Autodesk Fusion 360 part; units mm, degrees
(part 5 of 6)
  arc A231 (-66.3069, 126.4592) -> (-66.9633, 126.6319) centre (-66.7286, 126.1905) ccw
  line L58 (-66.9633, 126.6319) -> (-67.5372, 126.3268)
  arc A232 (-67.5372, 126.3268) -> (-67.761, 125.686) centre (-67.3025, 125.8853) ccw
  arc A233 (-68.3566, 123.3185) -> (-67.761, 125.686) centre (-69.5953, 124.8887) ccw
  arc A234 (-70.6799, 124.068) -> (-68.3566, 123.3185) centre (-69.0318, 125.2011) ccw
  arc A235 (-70.6799, 124.068) -> (-71.3419, 124.2178) centre (-71.0919, 123.7848) ccw
  line L59 (-71.3419, 124.2178) -> (-71.9048, 123.8928)
  arc A236 (-71.9048, 123.8928) -> (-72.1061, 123.2446) centre (-71.6548, 123.4598) ccw
  arc A237 (-72.6187, 120.8578) -> (-72.1061, 123.2446) centre (-73.9114, 122.3838) ccw
  arc A238 (-74.9667, 121.5258) -> (-72.6187, 120.8578) centre (-73.3592, 122.7156) ccw
  arc A239 (-74.9667, 121.5258) -> (-75.6336, 121.6523) centre (-75.3686, 121.2283) ccw
  line L60 (-75.6336, 121.6523) -> (-76.1848, 121.3079)
  arc A240 (-76.1848, 121.3079) -> (-76.3634, 120.653) centre (-75.9199, 120.8839) ccw
  arc A241 (-76.7923, 118.2498) -> (-76.3634, 120.653) centre (-78.1375, 119.7298) ccw
  arc A242 (-79.1623, 118.8354) -> (-76.7923, 118.2498) centre (-77.5972, 120.0807) ccw
  arc A243 (-79.1623, 118.8354) -> (-79.8331, 118.9387) centre (-79.5535, 118.5241) ccw
  line L61 (-79.8331, 118.9387) -> (-80.372, 118.5752)
  arc A244 (-80.372, 118.5752) -> (-80.5276, 117.9145) centre (-80.0924, 118.1607) ccw
  arc A245 (-80.8724, 115.4978) -> (-80.5276, 117.9145) centre (-82.2684, 116.9299) ccw
  arc A246 (-83.2613, 116.0003) -> (-80.8724, 115.4978) centre (-81.7407, 117.2994) ccw
  arc A247 (-83.2613, 116.0003) -> (-83.9354, 116.0801) centre (-83.6415, 115.6756) ccw
  line L62 (-83.9354, 116.0801) -> (-84.4612, 115.698)
  arc A248 (-84.4612, 115.698) -> (-84.5937, 115.0323) centre (-84.1673, 115.2935) ccw
  arc A249 (-84.8539, 112.605) -> (-84.5937, 115.0323) centre (-86.2991, 113.9875) ccw
  arc A250 (-87.259, 113.0239) -> (-84.8539, 112.605) centre (-85.7846, 114.3753) ccw
  arc A251 (-87.259, 113.0239) -> (-87.9354, 113.08) centre (-87.6276, 112.686) ccw
  line L63 (-87.9354, 113.08) -> (-88.4476, 112.6799)
  arc A252 (-88.4476, 112.6799) -> (-88.5567, 112.01) centre (-88.1398, 112.2859) ccw
  arc A253 (-88.7321, 109.575) -> (-88.5567, 112.01) centre (-90.2247, 110.9063) ccw
  arc A254 (-91.1503, 109.9097) -> (-88.7321, 109.575) centre (-89.724, 111.3118) ccw
  arc A255 (-91.1503, 109.9097) -> (-91.8283, 109.9423) centre (-91.5069, 109.5592) ccw
  line L64 (-91.8283, 109.9423) -> (-92.3262, 109.5244)
  arc A256 (-92.3262, 109.5244) -> (-92.4119, 108.8511) centre (-92.0048, 109.1414) ccw
  arc A257 (-92.5022, 106.4116) -> (-92.4119, 108.8511) centre (-94.0403, 107.6899) ccw
  arc A258 (-94.9306, 106.6617) -> (-92.5022, 106.4116) centre (-93.554, 108.1126) ccw
  arc A259 (-94.9306, 106.6617) -> (-95.6092, 106.6705) centre (-95.2747, 106.299) ccw
  line L65 (-95.6092, 106.6705) -> (-96.0923, 106.2356)
  arc A260 (-96.0923, 106.2356) -> (-96.1544, 105.5597) centre (-95.7577, 105.864) ccw
  arc A261 (-96.1595, 103.1185) -> (-96.1544, 105.5597) centre (-97.7413, 104.3424) ccw
  arc A262 (-98.5952, 103.2837) -> (-96.1595, 103.1185) centre (-97.2701, 104.7818) ccw
  arc A263 (-98.5952, 103.2837) -> (-99.2737, 103.2688) centre (-98.9264, 102.9092) ccw
  line L66 (-99.2737, 103.2688) -> (-99.7413, 102.8173)
  arc A264 (-99.7413, 102.8173) -> (-99.7798, 102.1396) centre (-99.394, 102.4576) ccw
  arc A265 (-99.6997, 99.6997) -> (-99.7798, 102.1396) centre (-101.3233, 100.8677) ccw
  arc A266 (-102.1396, 99.7798) -> (-99.6997, 99.6997) centre (-100.8677, 101.3233) ccw
  arc A267 (-102.1396, 99.7798) -> (-102.8173, 99.7413) centre (-102.4576, 99.394) ccw
  line L67 (-102.8173, 99.7413) -> (-103.2688, 99.2737)
  arc A268 (-103.2688, 99.2737) -> (-103.2837, 98.5952) centre (-102.9092, 98.9264) ccw
  arc A269 (-103.1185, 96.1595) -> (-103.2837, 98.5952) centre (-104.7818, 97.2701) ccw
  arc A270 (-105.5597, 96.1544) -> (-103.1185, 96.1595) centre (-104.3424, 97.7413) ccw
  arc A271 (-105.5597, 96.1544) -> (-106.2356, 96.0923) centre (-105.864, 95.7577) ccw
  line L68 (-106.2356, 96.0923) -> (-106.6705, 95.6092)
  arc A272 (-106.6705, 95.6092) -> (-106.6617, 94.9306) centre (-106.299, 95.2747) ccw
  arc A273 (-106.4116, 92.5022) -> (-106.6617, 94.9306) centre (-108.1126, 93.554) ccw
  arc A274 (-108.8511, 92.4119) -> (-106.4116, 92.5022) centre (-107.6899, 94.0403) ccw
  arc A275 (-108.8511, 92.4119) -> (-109.5244, 92.3262) centre (-109.1414, 92.0048) ccw
  line L69 (-109.5244, 92.3262) -> (-109.9423, 91.8283)
  arc A276 (-109.9423, 91.8283) -> (-109.9097, 91.1503) centre (-109.5592, 91.5069) ccw
  arc A277 (-109.575, 88.7321) -> (-109.9097, 91.1503) centre (-111.3118, 89.724) ccw
  arc A278 (-112.01, 88.5567) -> (-109.575, 88.7321) centre (-110.9063, 90.2247) ccw
  arc A279 (-112.01, 88.5567) -> (-112.6799, 88.4476) centre (-112.2859, 88.1398) ccw
  line L70 (-112.6799, 88.4476) -> (-113.08, 87.9354)
  arc A280 (-113.08, 87.9354) -> (-113.0239, 87.259) centre (-112.686, 87.6276) ccw
  arc A281 (-112.605, 84.8539) -> (-113.0239, 87.259) centre (-114.3753, 85.7846) ccw
  arc A282 (-115.0323, 84.5937) -> (-112.605, 84.8539) centre (-113.9875, 86.2991) ccw
  arc A283 (-115.0323, 84.5937) -> (-115.698, 84.4612) centre (-115.2935, 84.1673) ccw
  line L71 (-115.698, 84.4612) -> (-116.0801, 83.9354)
  arc A284 (-116.0801, 83.9354) -> (-116.0003, 83.2613) centre (-115.6756, 83.6415) ccw
  arc A285 (-115.4978, 80.8724) -> (-116.0003, 83.2613) centre (-117.2994, 81.7407) ccw
  arc A286 (-117.9145, 80.5276) -> (-115.4978, 80.8724) centre (-116.9299, 82.2684) ccw
  arc A287 (-117.9145, 80.5276) -> (-118.5752, 80.372) centre (-118.1607, 80.0924) ccw
  line L72 (-118.5752, 80.372) -> (-118.9387, 79.8331)
  arc A288 (-118.9387, 79.8331) -> (-118.8354, 79.1623) centre (-118.5241, 79.5535) ccw
  arc A289 (-118.2498, 76.7923) -> (-118.8354, 79.1623) centre (-120.0807, 77.5972) ccw
  arc A290 (-120.653, 76.3634) -> (-118.2498, 76.7923) centre (-119.7298, 78.1375) ccw
  arc A291 (-120.653, 76.3634) -> (-121.3079, 76.1848) centre (-120.8839, 75.9199) ccw
  line L73 (-121.3079, 76.1848) -> (-121.6523, 75.6336)
  arc A292 (-121.6523, 75.6336) -> (-121.5258, 74.9667) centre (-121.2283, 75.3686) ccw
  arc A293 (-120.8578, 72.6187) -> (-121.5258, 74.9667) centre (-122.7156, 73.3592) ccw
  arc A294 (-123.2446, 72.1061) -> (-120.8578, 72.6187) centre (-122.3838, 73.9114) ccw
  arc A295 (-123.2446, 72.1061) -> (-123.8928, 71.9048) centre (-123.4598, 71.6548) ccw
  line L74 (-123.8928, 71.9048) -> (-124.2178, 71.3419)
  arc A296 (-124.2178, 71.3419) -> (-124.068, 70.6799) centre (-123.7848, 71.0919) ccw
  arc A297 (-123.3185, 68.3566) -> (-124.068, 70.6799) centre (-125.2011, 69.0318) ccw
  arc A298 (-125.686, 67.761) -> (-123.3185, 68.3566) centre (-124.8887, 69.5953) ccw
  arc A299 (-125.686, 67.761) -> (-126.3268, 67.5372) centre (-125.8853, 67.3025) ccw
  line L75 (-126.3268, 67.5372) -> (-126.6319, 66.9633)
  arc A300 (-126.6319, 66.9633) -> (-126.4592, 66.3069) centre (-126.1905, 66.7286) ccw
  arc A301 (-125.629, 64.0112) -> (-126.4592, 66.3069) centre (-127.534, 64.6203) ccw
  arc A302 (-127.9742, 63.3334) -> (-125.629, 64.0112) centre (-127.2415, 65.1943) ccw
  arc A303 (-127.9742, 63.3334) -> (-128.6068, 63.0873) centre (-128.1574, 62.8682) ccw
  line L76 (-128.6068, 63.0873) -> (-128.8918, 62.5031)
  arc A304 (-128.8918, 62.5031) -> (-128.6962, 61.8532) centre (-128.4424, 62.2839) ccw
  arc A305 (-127.7864, 59.5878) -> (-128.6962, 61.8532) centre (-129.7115, 60.13) ccw
  arc A306 (-130.1066, 58.8286) -> (-127.7864, 59.5878) centre (-129.4392, 60.7139) ccw
  arc A307 (-130.1066, 58.8286) -> (-130.7302, 58.5606) centre (-130.2734, 58.3572) ccw
  line L77 (-130.7302, 58.5606) -> (-130.9946, 57.9668)
  arc A308 (-130.9946, 57.9668) -> (-130.7764, 57.324) centre (-130.5378, 57.7634) ccw
  arc A309 (-129.7882, 55.0918) -> (-130.7764, 57.324) centre (-131.731, 55.5665) ccw
  arc A310 (-132.0804, 54.2521) -> (-129.7882, 55.0918) centre (-131.4793, 56.1596) ccw
  arc A311 (-132.0804, 54.2521) -> (-132.6943, 53.9625) centre (-132.2307, 53.7752) ccw
  line L78 (-132.6943, 53.9625) -> (-132.9378, 53.3598)
  arc A312 (-132.9378, 53.3598) -> (-132.6974, 52.7251) centre (-132.4742, 53.1725) ccw
  arc A313 (-131.6318, 50.5287) -> (-132.6974, 52.7251) centre (-133.59, 50.9353) ccw
  arc A314 (-133.8933, 49.6095) -> (-131.6318, 50.5287) centre (-133.3591, 51.5368) ccw
  arc A315 (-133.8933, 49.6095) -> (-134.4967, 49.2987) centre (-134.0269, 49.1277) ccw
  line L79 (-134.4967, 49.2987) -> (-134.719, 48.6879)
  arc A316 (-134.719, 48.6879) -> (-134.4566, 48.0619) centre (-134.2492, 48.5169) ccw
  arc A317 (-133.315, 45.904) -> (-134.4566, 48.0619) centre (-135.2862, 46.2421) ccw
  arc A318 (-135.5431, 44.9065) -> (-133.315, 45.904) centre (-135.0765, 46.8513) ccw
  arc A319 (-135.5431, 44.9065) -> (-136.1353, 44.5748) centre (-135.6598, 44.4203) ccw
  line L80 (-136.1353, 44.5748) -> (-136.3362, 43.9566)
  arc A320 (-136.3362, 43.9566) -> (-136.052, 43.3402) centre (-135.8606, 43.8021) ccw
  arc A321 (-134.8358, 41.2235) -> (-136.052, 43.3402) centre (-136.8177, 41.4925) ccw
  arc A322 (-137.0278, 40.1487) -> (-134.8358, 41.2235) centre (-136.6293, 42.1086) ccw
  arc A323 (-137.0278, 40.1487) -> (-137.608, 39.7966) centre (-137.1274, 39.6587) ccw
  line L81 (-137.608, 39.7966) -> (-137.7872, 39.1717)
  arc A324 (-137.7872, 39.1717) -> (-137.4817, 38.5656) centre (-137.3065, 39.0339) ccw
  arc A325 (-136.1924, 36.4926) -> (-137.4817, 38.5656) centre (-138.1824, 36.6924) ccw
  arc A326 (-138.3455, 35.3421) -> (-136.1924, 36.4926) centre (-138.0156, 37.3147) ccw
  arc A327 (-138.3455, 35.3421) -> (-138.9131, 34.9699) centre (-138.4279, 34.8489) ccw
  line L82 (-138.9131, 34.9699) -> (-139.0703, 34.3392)
  arc A328 (-139.0703, 34.3392) -> (-138.7439, 33.7441) centre (-138.5852, 34.2182) ccw
  arc A329 (-137.383, 31.7174) -> (-138.7439, 33.7441) centre (-139.3787, 31.8475) ccw
  arc A330 (-139.4946, 30.4923) -> (-137.383, 31.7174) centre (-139.2338, 32.4753) ccw
  arc A331 (-139.4946, 30.4923) -> (-140.0489, 30.1006) centre (-139.5598, 29.9966) ccw
  line L83 (-140.0489, 30.1006) -> (-140.184, 29.4648)
  arc A332 (-140.184, 29.4648) -> (-139.837, 28.8814) centre (-139.6949, 29.3608) ccw
  arc A333 (-138.4062, 26.9034) -> (-139.837, 28.8814) centre (-140.4053, 26.9639) ccw
  arc A334 (-140.4738, 25.6055) -> (-138.4062, 26.9034) centre (-140.2824, 27.5963) ccw
  arc A335 (-140.4738, 25.6055) -> (-141.014, 25.1946) centre (-140.5216, 25.1078) ccw
  line L84 (-141.014, 25.1946) -> (-141.1269, 24.5545)
  arc A336 (-141.1269, 24.5545) -> (-140.7598, 23.9836) centre (-140.6345, 24.4676) ccw
  arc A337 (-139.2608, 22.0567) -> (-140.7598, 23.9836) centre (-141.2608, 22.0474) ccw
  arc A338 (-141.2818, 20.6874) -> (-139.2608, 22.0567) centre (-141.16, 22.6837) ccw
  arc A339 (-141.2818, 20.6874) -> (-141.8074, 20.2579) centre (-141.3123, 20.1883) ccw
  line L85 (-141.8074, 20.2579) -> (-141.8979, 19.6143)
  arc A340 (-141.8979, 19.6143) -> (-141.511, 19.0565) centre (-141.4028, 19.5447) ccw
  arc A341 (-139.9458, 17.1832) -> (-141.511, 19.0565) centre (-141.9442, 17.104) ccw
  arc A342 (-141.9177, 15.7441) -> (-139.9458, 17.1832) centre (-141.8657, 17.7435) ccw
  arc A343 (-141.9177, 15.7441) -> (-142.428, 15.2966) centre (-141.9308, 15.2443) ccw
  line L86 (-142.428, 15.2966) -> (-142.496, 14.6501)
  arc A344 (-142.496, 14.6501) -> (-142.0899, 14.1063) centre (-141.9987, 14.5979) ccw
  arc A345 (-140.4602, 12.2887) -> (-142.0899, 14.1063) centre (-142.4546, 12.1398) ccw
  arc A346 (-142.3808, 10.7817) -> (-140.4602, 12.2887) centre (-142.3985, 12.7816) ccw
  arc A347 (-142.3808, 10.7817) -> (-142.8751, 10.3166) centre (-142.3763, 10.2817) ccw
  line L87 (-142.8751, 10.3166) -> (-142.9205, 9.6682)
  arc A348 (-142.9205, 9.6682) -> (-142.4956, 9.1388) centre (-142.4217, 9.6333) ccw
  arc A349 (-140.8035, 7.3792) -> (-142.4956, 9.1388) centre (-142.7915, 7.1608) ccw
  arc A350 (-142.6703, 5.8061) -> (-140.8035, 7.3792) centre (-142.7578, 7.8042) ccw
  arc A351 (-142.6703, 5.8061) -> (-143.1481, 5.324) centre (-142.6484, 5.3066) ccw
  line L88 (-143.1481, 5.324) -> (-143.1708, 4.6744)
  arc A352 (-143.1708, 4.6744) -> (-142.7278, 4.1602) centre (-142.6711, 4.657) ccw
  arc A353 (-140.9752, 2.4607) -> (-142.7278, 4.1602) centre (-142.9545, 2.1731) ccw
  arc A354 (-142.786, 0.8235) -> (-140.9752, 2.4607) centre (-142.9432, 2.8173) ccw
  arc A355 (-142.786, 0.8235) -> (-143.2467, 0.325) centre (-142.7467, 0.325) ccw
  line L89 (-143.2467, 0.325) -> (-143.2467, -0.325)
  arc A356 (-143.2467, -0.325) -> (-142.786, -0.8235) centre (-142.7467, -0.325) ccw
  arc A357 (-140.9752, -2.4607) -> (-142.786, -0.8235) centre (-142.9432, -2.8173) ccw
  arc A358 (-142.7278, -4.1602) -> (-140.9752, -2.4607) centre (-142.9545, -2.1731) ccw
  arc A359 (-142.7278, -4.1602) -> (-143.1708, -4.6744) centre (-142.6711, -4.657) ccw
  line L90 (-143.1708, -4.6744) -> (-143.1481, -5.324)
  arc A360 (-143.1481, -5.324) -> (-142.6703, -5.8061) centre (-142.6484, -5.3066) ccw
  arc A361 (-140.8035, -7.3792) -> (-142.6703, -5.8061) centre (-142.7578, -7.8042) ccw
  arc A362 (-142.4956, -9.1388) -> (-140.8035, -7.3792) centre (-142.7915, -7.1608) ccw
  arc A363 (-142.4956, -9.1388) -> (-142.9205, -9.6682) centre (-142.4217, -9.6333) ccw
  line L91 (-142.9205, -9.6682) -> (-142.8751, -10.3166)
  arc A364 (-142.8751, -10.3166) -> (-142.3808, -10.7817) centre (-142.3763, -10.2817) ccw
  arc A365 (-140.4602, -12.2887) -> (-142.3808, -10.7817) centre (-142.3985, -12.7816) ccw
  arc A366 (-142.0899, -14.1063) -> (-140.4602, -12.2887) centre (-142.4546, -12.1398) ccw
  arc A367 (-142.0899, -14.1063) -> (-142.496, -14.6501) centre (-141.9987, -14.5979) ccw
  line L92 (-142.496, -14.6501) -> (-142.428, -15.2966)
  arc A368 (-142.428, -15.2966) -> (-141.9177, -15.7441) centre (-141.9308, -15.2443) ccw
  arc A369 (-139.9458, -17.1832) -> (-141.9177, -15.7441) centre (-141.8657, -17.7435) ccw
  arc A370 (-141.511, -19.0565) -> (-139.9458, -17.1832) centre (-141.9442, -17.104) ccw
  arc A371 (-141.511, -19.0565) -> (-141.8979, -19.6143) centre (-141.4028, -19.5447) ccw
  line L93 (-141.8979, -19.6143) -> (-141.8074, -20.2579)
  arc A372 (-141.8074, -20.2579) -> (-141.2818, -20.6874) centre (-141.3123, -20.1883) ccw
  arc A373 (-139.2608, -22.0567) -> (-141.2818, -20.6874) centre (-141.16, -22.6837) ccw
  arc A374 (-140.7598, -23.9836) -> (-139.2608, -22.0567) centre (-141.2608, -22.0474) ccw
  arc A375 (-140.7598, -23.9836) -> (-141.1269, -24.5545) centre (-140.6345, -24.4676) ccw
  line L94 (-141.1269, -24.5545) -> (-141.014, -25.1946)
  arc A376 (-141.014, -25.1946) -> (-140.4738, -25.6055) centre (-140.5216, -25.1078) ccw
  arc A377 (-138.4062, -26.9034) -> (-140.4738, -25.6055) centre (-140.2824, -27.5963) ccw
  arc A378 (-139.837, -28.8814) -> (-138.4062, -26.9034) centre (-140.4053, -26.9639) ccw
  arc A379 (-139.837, -28.8814) -> (-140.184, -29.4648) centre (-139.6949, -29.3608) ccw
  line L95 (-140.184, -29.4648) -> (-140.0489, -30.1006)
  arc A380 (-140.0489, -30.1006) -> (-139.4946, -30.4923) centre (-139.5598, -29.9966) ccw
  arc A381 (-137.383, -31.7174) -> (-139.4946, -30.4923) centre (-139.2338, -32.4753) ccw
  arc A382 (-138.7439, -33.7441) -> (-137.383, -31.7174) centre (-139.3787, -31.8475) ccw
  arc A383 (-138.7439, -33.7441) -> (-139.0703, -34.3392) centre (-138.5852, -34.2182) ccw
  line L96 (-139.0703, -34.3392) -> (-138.9131, -34.9699)
  arc A384 (-138.9131, -34.9699) -> (-138.3455, -35.3421) centre (-138.4279, -34.8489) ccw
  arc A385 (-136.1924, -36.4926) -> (-138.3455, -35.3421) centre (-138.0156, -37.3147) ccw
  arc A386 (-137.4817, -38.5656) -> (-136.1924, -36.4926) centre (-138.1824, -36.6924) ccw
  arc A387 (-137.4817, -38.5656) -> (-137.7872, -39.1717) centre (-137.3065, -39.0339) ccw
  line L97 (-137.7872, -39.1717) -> (-137.608, -39.7966)
  arc A388 (-137.608, -39.7966) -> (-137.0278, -40.1487) centre (-137.1274, -39.6587) ccw
  arc A389 (-134.8358, -41.2235) -> (-137.0278, -40.1487) centre (-136.6293, -42.1086) ccw
  arc A390 (-136.052, -43.3402) -> (-134.8358, -41.2235) centre (-136.8177, -41.4925) ccw
  arc A391 (-136.052, -43.3402) -> (-136.3362, -43.9566) centre (-135.8606, -43.8021) ccw
  line L98 (-136.3362, -43.9566) -> (-136.1353, -44.5748)
  arc A392 (-136.1353, -44.5748) -> (-135.5431, -44.9065) centre (-135.6598, -44.4203) ccw
  arc A393 (-133.315, -45.904) -> (-135.5431, -44.9065) centre (-135.0765, -46.8513) ccw
  arc A394 (-134.4566, -48.0619) -> (-133.315, -45.904) centre (-135.2862, -46.2421) ccw
  arc A395 (-134.4566, -48.0619) -> (-134.719, -48.6879) centre (-134.2492, -48.5169) ccw
  line L99 (-134.719, -48.6879) -> (-134.4967, -49.2987)
  arc A396 (-134.4967, -49.2987) -> (-133.8933, -49.6095) centre (-134.0269, -49.1277) ccw
  arc A397 (-131.6318, -50.5287) -> (-133.8933, -49.6095) centre (-133.3591, -51.5368) ccw
  arc A398 (-132.6974, -52.7251) -> (-131.6318, -50.5287) centre (-133.59, -50.9353) ccw
  arc A399 (-132.6974, -52.7251) -> (-132.9378, -53.3598) centre (-132.4742, -53.1725) ccw
  line L100 (-132.9378, -53.3598) -> (-132.6943, -53.9625)
  arc A400 (-132.6943, -53.9625) -> (-132.0804, -54.2521) centre (-132.2307, -53.7752) ccw
  arc A401 (-129.7882, -55.0918) -> (-132.0804, -54.2521) centre (-131.4793, -56.1596) ccw
  arc A402 (-130.7764, -57.324) -> (-129.7882, -55.0918) centre (-131.731, -55.5665) ccw
  arc A403 (-130.7764, -57.324) -> (-130.9946, -57.9668) centre (-130.5378, -57.7634) ccw
  line L101 (-130.9946, -57.9668) -> (-130.7302, -58.5606)
  arc A404 (-130.7302, -58.5606) -> (-130.1066, -58.8286) centre (-130.2734, -58.3572) ccw
  arc A405 (-127.7864, -59.5878) -> (-130.1066, -58.8286) centre (-129.4392, -60.7139) ccw
  arc A406 (-128.6962, -61.8532) -> (-127.7864, -59.5878) centre (-129.7115, -60.13) ccw
  arc A407 (-128.6962, -61.8532) -> (-128.8918, -62.5031) centre (-128.4424, -62.2839) ccw
  line L102 (-128.8918, -62.5031) -> (-128.6068, -63.0873)
  arc A408 (-128.6068, -63.0873) -> (-127.9742, -63.3334) centre (-128.1574, -62.8682) ccw
  arc A409 (-125.629, -64.0112) -> (-127.9742, -63.3334) centre (-127.2415, -65.1943) ccw
  arc A410 (-126.4592, -66.3069) -> (-125.629, -64.0112) centre (-127.534, -64.6203) ccw
  arc A411 (-126.4592, -66.3069) -> (-126.6319, -66.9633) centre (-126.1905, -66.7286) ccw
  line L103 (-126.6319, -66.9633) -> (-126.3268, -67.5372)
  arc A412 (-126.3268, -67.5372) -> (-125.686, -67.761) centre (-125.8853, -67.3025) ccw
  arc A413 (-123.3185, -68.3566) -> (-125.686, -67.761) centre (-124.8887, -69.5953) ccw
  arc A414 (-124.068, -70.6799) -> (-123.3185, -68.3566) centre (-125.2011, -69.0318) ccw
  arc A415 (-124.068, -70.6799) -> (-124.2178, -71.3419) centre (-123.7848, -71.0919) ccw
  line L104 (-124.2178, -71.3419) -> (-123.8928, -71.9048)
  arc A416 (-123.8928, -71.9048) -> (-123.2446, -72.1061) centre (-123.4598, -71.6548) ccw
  arc A417 (-120.8578, -72.6187) -> (-123.2446, -72.1061) centre (-122.3838, -73.9114) ccw
  arc A418 (-121.5258, -74.9667) -> (-120.8578, -72.6187) centre (-122.7156, -73.3592) ccw
  arc A419 (-121.5258, -74.9667) -> (-121.6523, -75.6336) centre (-121.2283, -75.3686) ccw
  line L105 (-121.6523, -75.6336) -> (-121.3079, -76.1848)
  arc A420 (-121.3079, -76.1848) -> (-120.653, -76.3634) centre (-120.8839, -75.9199) ccw
  arc A421 (-118.2498, -76.7923) -> (-120.653, -76.3634) centre (-119.7298, -78.1375) ccw
  arc A422 (-118.8354, -79.1623) -> (-118.2498, -76.7923) centre (-120.0807, -77.5972) ccw
  arc A423 (-118.8354, -79.1623) -> (-118.9387, -79.8331) centre (-118.5241, -79.5535) ccw
  line L106 (-118.9387, -79.8331) -> (-118.5752, -80.372)
  arc A424 (-118.5752, -80.372) -> (-117.9145, -80.5276) centre (-118.1607, -80.0924) ccw
  arc A425 (-115.4978, -80.8724) -> (-117.9145, -80.5276) centre (-116.9299, -82.2684) ccw
  arc A426 (-116.0003, -83.2613) -> (-115.4978, -80.8724) centre (-117.2994, -81.7407) ccw
  arc A427 (-116.0003, -83.2613) -> (-116.0801, -83.9354) centre (-115.6756, -83.6415) ccw
  line L107 (-116.0801, -83.9354) -> (-115.698, -84.4612)
  arc A428 (-115.698, -84.4612) -> (-115.0323, -84.5937) centre (-115.2935, -84.1673) ccw
  arc A429 (-112.605, -84.8539) -> (-115.0323, -84.5937) centre (-113.9875, -86.2991) ccw
  arc A430 (-113.0239, -87.259) -> (-112.605, -84.8539) centre (-114.3753, -85.7846) ccw
  arc A431 (-113.0239, -87.259) -> (-113.08, -87.9354) centre (-112.686, -87.6276) ccw
  line L108 (-113.08, -87.9354) -> (-112.6799, -88.4476)
  arc A432 (-112.6799, -88.4476) -> (-112.01, -88.5567) centre (-112.2859, -88.1398) ccw
  arc A433 (-109.575, -88.7321) -> (-112.01, -88.5567) centre (-110.9063, -90.2247) ccw
  arc A434 (-109.9097, -91.1503) -> (-109.575, -88.7321) centre (-111.3118, -89.724) ccw
  arc A435 (-109.9097, -91.1503) -> (-109.9423, -91.8283) centre (-109.5592, -91.5069) ccw
  line L109 (-109.9423, -91.8283) -> (-109.5244, -92.3262)
  arc A436 (-109.5244, -92.3262) -> (-108.8511, -92.4119) centre (-109.1414, -92.0048) ccw
  arc A437 (-106.4116, -92.5022) -> (-108.8511, -92.4119) centre (-107.6899, -94.0403) ccw
  arc A438 (-106.6617, -94.9306) -> (-106.4116, -92.5022) centre (-108.1126, -93.554) ccw
  arc A439 (-106.6617, -94.9306) -> (-106.6705, -95.6092) centre (-106.299, -95.2747) ccw
  line L110 (-106.6705, -95.6092) -> (-106.2356, -96.0923)
  arc A440 (-106.2356, -96.0923) -> (-105.5597, -96.1544) centre (-105.864, -95.7577) ccw
  arc A441 (-103.1185, -96.1595) -> (-105.5597, -96.1544) centre (-104.3424, -97.7413) ccw
  arc A442 (-103.2837, -98.5952) -> (-103.1185, -96.1595) centre (-104.7818, -97.2701) ccw
  arc A443 (-103.2837, -98.5952) -> (-103.2688, -99.2737) centre (-102.9092, -98.9264) ccw
  line L111 (-103.2688, -99.2737) -> (-102.8173, -99.7413)
  arc A444 (-102.8173, -99.7413) -> (-102.1396, -99.7798) centre (-102.4576, -99.394) ccw
  arc A445 (-99.6997, -99.6997) -> (-102.1396, -99.7798) centre (-100.8677, -101.3233) ccw
  arc A446 (-99.7798, -102.1396) -> (-99.6997, -99.6997) centre (-101.3233, -100.8677) ccw
  arc A447 (-99.7798, -102.1396) -> (-99.7413, -102.8173) centre (-99.394, -102.4576) ccw
  line L112 (-99.7413, -102.8173) -> (-99.2737, -103.2688)
  arc A448 (-99.2737, -103.2688) -> (-98.5952, -103.2837) centre (-98.9264, -102.9092) ccw
  arc A449 (-96.1595, -103.1185) -> (-98.5952, -103.2837) centre (-97.2701, -104.7818) ccw
  arc A450 (-96.1544, -105.5597) -> (-96.1595, -103.1185) centre (-97.7413, -104.3424) ccw
  arc A451 (-96.1544, -105.5597) -> (-96.0923, -106.2356) centre (-95.7577, -105.864) ccw
  line L113 (-96.0923, -106.2356) -> (-95.6092, -106.6705)
  arc A452 (-95.6092, -106.6705) -> (-94.9306, -106.6617) centre (-95.2747, -106.299) ccw
  arc A453 (-92.5022, -106.4116) -> (-94.9306, -106.6617) centre (-93.554, -108.1126) ccw
  arc A454 (-92.4119, -108.8511) -> (-92.5022, -106.4116) centre (-94.0403, -107.6899) ccw
  arc A455 (-92.4119, -108.8511) -> (-92.3262, -109.5244) centre (-92.0048, -109.1414) ccw
  line L114 (-92.3262, -109.5244) -> (-91.8283, -109.9423)
  arc A456 (-91.8283, -109.9423) -> (-91.1503, -109.9097) centre (-91.5069, -109.5592) ccw
  arc A457 (-88.7321, -109.575) -> (-91.1503, -109.9097) centre (-89.724, -111.3118) ccw
  arc A458 (-88.5567, -112.01) -> (-88.7321, -109.575) centre (-90.2247, -110.9063) ccw
  arc A459 (-88.5567, -112.01) -> (-88.4476, -112.6799) centre (-88.1398, -112.2859) ccw
  line L115 (-88.4476, -112.6799) -> (-87.9354, -113.08)
  arc A460 (-87.9354, -113.08) -> (-87.259, -113.0239) centre (-87.6276, -112.686) ccw
  arc A461 (-84.8539, -112.605) -> (-87.259, -113.0239) centre (-85.7846, -114.3753) ccw
  arc A462 (-84.5937, -115.0323) -> (-84.8539, -112.605) centre (-86.2991, -113.9875) ccw
  arc A463 (-84.5937, -115.0323) -> (-84.4612, -115.698) centre (-84.1673, -115.2935) ccw
  line L116 (-84.4612, -115.698) -> (-83.9354, -116.0801)
  arc A464 (-83.9354, -116.0801) -> (-83.2613, -116.0003) centre (-83.6415, -115.6756) ccw
  arc A465 (-80.8724, -115.4978) -> (-83.2613, -116.0003) centre (-81.7407, -117.2994) ccw
  arc A466 (-80.5276, -117.9145) -> (-80.8724, -115.4978) centre (-82.2684, -116.9299) ccw
  arc A467 (-80.5276, -117.9145) -> (-80.372, -118.5752) centre (-80.0924, -118.1607) ccw
  line L117 (-80.372, -118.5752) -> (-79.8331, -118.9387)
  arc A468 (-79.8331, -118.9387) -> (-79.1623, -118.8354) centre (-79.5535, -118.5241) ccw
  arc A469 (-76.7923, -118.2498) -> (-79.1623, -118.8354) centre (-77.5972, -120.0807) ccw
  arc A470 (-76.3634, -120.653) -> (-76.7923, -118.2498) centre (-78.1375, -119.7298) ccw
  arc A471 (-76.3634, -120.653) -> (-76.1848, -121.3079) centre (-75.9199, -120.8839) ccw
  line L118 (-76.1848, -121.3079) -> (-75.6336, -121.6523)
  arc A472 (-75.6336, -121.6523) -> (-74.9667, -121.5258) centre (-75.3686, -121.2283) ccw
  arc A473 (-72.6187, -120.8578) -> (-74.9667, -121.5258) centre (-73.3592, -122.7156) ccw
  arc A474 (-72.1061, -123.2446) -> (-72.6187, -120.8578) centre (-73.9114, -122.3838) ccw
  arc A475 (-72.1061, -123.2446) -> (-71.9048, -123.8928) centre (-71.6548, -123.4598) ccw
  line L119 (-71.9048, -123.8928) -> (-71.3419, -124.2178)
  arc A476 (-71.3419, -124.2178) -> (-70.6799, -124.068) centre (-71.0919, -123.7848) ccw
  arc A477 (-68.3566, -123.3185) -> (-70.6799, -124.068) centre (-69.0318, -125.2011) ccw
  arc A478 (-67.761, -125.686) -> (-68.3566, -123.3185) centre (-69.5953, -124.8887) ccw
  arc A479 (-67.761, -125.686) -> (-67.5372, -126.3268) centre (-67.3025, -125.8853) ccw
  line L120 (-67.5372, -126.3268) -> (-66.9633, -126.6319)
  arc A480 (-66.9633, -126.6319) -> (-66.3069, -126.4592) centre (-66.7286, -126.1905) ccw
  arc A481 (-64.0112, -125.629) -> (-66.3069, -126.4592) centre (-64.6203, -127.534) ccw
  arc A482 (-63.3334, -127.9742) -> (-64.0112, -125.629) centre (-65.1943, -127.2415) ccw
  arc A483 (-63.3334, -127.9742) -> (-63.0873, -128.6068) centre (-62.8682, -128.1574) ccw
  line L121 (-63.0873, -128.6068) -> (-62.5031, -128.8918)
  arc A484 (-62.5031, -128.8918) -> (-61.8532, -128.6962) centre (-62.2839, -128.4424) ccw
  arc A485 (-59.5878, -127.7864) -> (-61.8532, -128.6962) centre (-60.13, -129.7115) ccw
  arc A486 (-58.8286, -130.1066) -> (-59.5878, -127.7864) centre (-60.7139, -129.4392) ccw
  arc A487 (-58.8286, -130.1066) -> (-58.5606, -130.7302) centre (-58.3572, -130.2734) ccw
  line L122 (-58.5606, -130.7302) -> (-57.9668, -130.9946)
  arc A488 (-57.9668, -130.9946) -> (-57.324, -130.7764) centre (-57.7634, -130.5378) ccw
  arc A489 (-55.0918, -129.7882) -> (-57.324, -130.7764) centre (-55.5665, -131.731) ccw
  arc A490 (-54.2521, -132.0804) -> (-55.0918, -129.7882) centre (-56.1596, -131.4793) ccw
  arc A491 (-54.2521, -132.0804) -> (-53.9625, -132.6943) centre (-53.7752, -132.2307) ccw
  line L123 (-53.9625, -132.6943) -> (-53.3598, -132.9378)
  arc A492 (-53.3598, -132.9378) -> (-52.7251, -132.6974) centre (-53.1725, -132.4742) ccw
  arc A493 (-50.5287, -131.6318) -> (-52.7251, -132.6974) centre (-50.9353, -133.59) ccw
  arc A494 (-49.6095, -133.8933) -> (-50.5287, -131.6318) centre (-51.5368, -133.3591) ccw
  arc A495 (-49.6095, -133.8933) -> (-49.2987, -134.4967) centre (-49.1277, -134.0269) ccw
  line L124 (-49.2987, -134.4967) -> (-48.6879, -134.719)
  arc A496 (-48.6879, -134.719) -> (-48.0619, -134.4566) centre (-48.5169, -134.2492) ccw
  arc A497 (-45.904, -133.315) -> (-48.0619, -134.4566) centre (-46.2421, -135.2862) ccw
  arc A498 (-44.9065, -135.5431) -> (-45.904, -133.315) centre (-46.8513, -135.0765) ccw
  arc A499 (-44.9065, -135.5431) -> (-44.5748, -136.1353) centre (-44.4203, -135.6598) ccw
  line L125 (-44.5748, -136.1353) -> (-43.9566, -136.3362)
  arc A500 (-43.9566, -136.3362) -> (-43.3402, -136.052) centre (-43.8021, -135.8606) ccw
  arc A501 (-41.2235, -134.8358) -> (-43.3402, -136.052) centre (-41.4925, -136.8177) ccw
  arc A502 (-40.1487, -137.0278) -> (-41.2235, -134.8358) centre (-42.1086, -136.6293) ccw
  arc A503 (-40.1487, -137.0278) -> (-39.7966, -137.608) centre (-39.6587, -137.1274) ccw
  line L126 (-39.7966, -137.608) -> (-39.1717, -137.7872)
  arc A504 (-39.1717, -137.7872) -> (-38.5656, -137.4817) centre (-39.0339, -137.3065) ccw
  arc A505 (-36.4926, -136.1924) -> (-38.5656, -137.4817) centre (-36.6924, -138.1824) ccw
  arc A506 (-35.3421, -138.3455) -> (-36.4926, -136.1924) centre (-37.3147, -138.0156) ccw
  arc A507 (-35.3421, -138.3455) -> (-34.9699, -138.9131) centre (-34.8489, -138.4279) ccw
  line L127 (-34.9699, -138.9131) -> (-34.3392, -139.0703)
  arc A508 (-34.3392, -139.0703) -> (-33.7441, -138.7439) centre (-34.2182, -138.5852) ccw
  arc A509 (-31.7174, -137.383) -> (-33.7441, -138.7439) centre (-31.8475, -139.3787) ccw
  arc A510 (-30.4923, -139.4946) -> (-31.7174, -137.383) centre (-32.4753, -139.2338) ccw
  arc A511 (-30.4923, -139.4946) -> (-30.1006, -140.0489) centre (-29.9966, -139.5598) ccw
  line L128 (-30.1006, -140.0489) -> (-29.4648, -140.184)
  arc A512 (-29.4648, -140.184) -> (-28.8814, -139.837) centre (-29.3608, -139.6949) ccw
  arc A513 (-26.9034, -138.4062) -> (-28.8814, -139.837) centre (-26.9639, -140.4053) ccw
  arc A514 (-25.6055, -140.4738) -> (-26.9034, -138.4062) centre (-27.5963, -140.2824) ccw
  arc A515 (-25.6055, -140.4738) -> (-25.1946, -141.014) centre (-25.1078, -140.5216) ccw
  line L129 (-25.1946, -141.014) -> (-24.5545, -141.1269)
  arc A516 (-24.5545, -141.1269) -> (-23.9836, -140.7598) centre (-24.4676, -140.6345) ccw
  arc A517 (-22.0567, -139.2608) -> (-23.9836, -140.7598) centre (-22.0474, -141.2608) ccw
  arc A518 (-20.6874, -141.2818) -> (-22.0567, -139.2608) centre (-22.6837, -141.16) ccw
  arc A519 (-20.6874, -141.2818) -> (-20.2579, -141.8074) centre (-20.1883, -141.3123) ccw
  line L130 (-20.2579, -141.8074) -> (-19.6143, -141.8979)
  arc A520 (-19.6143, -141.8979) -> (-19.0565, -141.511) centre (-19.5447, -141.4028) ccw
  arc A521 (-17.1832, -139.9458) -> (-19.0565, -141.511) centre (-17.104, -141.9442) ccw
  arc A522 (-15.7441, -141.9177) -> (-17.1832, -139.9458) centre (-17.7435, -141.8657) ccw
  arc A523 (-15.7441, -141.9177) -> (-15.2966, -142.428) centre (-15.2443, -141.9308) ccw
  line L131 (-15.2966, -142.428) -> (-14.6501, -142.496)
  arc A524 (-14.6501, -142.496) -> (-14.1063, -142.0899) centre (-14.5979, -141.9987) ccw
  arc A525 (-12.2887, -140.4602) -> (-14.1063, -142.0899) centre (-12.1398, -142.4546) ccw
  arc A526 (-10.7817, -142.3808) -> (-12.2887, -140.4602) centre (-12.7816, -142.3985) ccw
  arc A527 (-10.7817, -142.3808) -> (-10.3166, -142.8751) centre (-10.2817, -142.3763) ccw
  line L132 (-10.3166, -142.8751) -> (-9.6682, -142.9205)
  arc A528 (-9.6682, -142.9205) -> (-9.1388, -142.4956) centre (-9.6333, -142.4217) ccw
  arc A529 (-7.3792, -140.8035) -> (-9.1388, -142.4956) centre (-7.1608, -142.7915) ccw
  arc A530 (-5.8061, -142.6703) -> (-7.3792, -140.8035) centre (-7.8042, -142.7578) ccw
  arc A531 (-5.8061, -142.6703) -> (-5.324, -143.1481) centre (-5.3066, -142.6484) ccw
  line L133 (-5.324, -143.1481) -> (-4.6744, -143.1708)
  arc A532 (-4.6744, -143.1708) -> (-4.1602, -142.7278) centre (-4.657, -142.6711) ccw
  arc A533 (-2.4607, -140.9752) -> (-4.1602, -142.7278) centre (-2.1731, -142.9545) ccw
  arc A534 (-0.8235, -142.786) -> (-2.4607, -140.9752) centre (-2.8173, -142.9432) ccw
  arc A535 (-0.8235, -142.786) -> (-0.325, -143.2467) centre (-0.325, -142.7467) ccw
  line L134 (-0.325, -143.2467) -> (0.325, -143.2467)
  arc A536 (0.325, -143.2467) -> (0.8235, -142.786) centre (0.325, -142.7467) ccw
  arc A537 (2.4607, -140.9752) -> (0.8235, -142.786) centre (2.8173, -142.9432) ccw
  arc A538 (4.1602, -142.7278) -> (2.4607, -140.9752) centre (2.1731, -142.9545) ccw
  arc A539 (4.1602, -142.7278) -> (4.6744, -143.1708) centre (4.657, -142.6711) ccw
  line L135 (4.6744, -143.1708) -> (5.324, -143.1481)
  arc A540 (5.324, -143.1481) -> (5.8061, -142.6703) centre (5.3066, -142.6484) ccw
  arc A541 (7.3792, -140.8035) -> (5.8061, -142.6703) centre (7.8042, -142.7578) ccw
  arc A542 (9.1388, -142.4956) -> (7.3792, -140.8035) centre (7.1608, -142.7915) ccw
  arc A543 (9.1388, -142.4956) -> (9.6682, -142.9205) centre (9.6333, -142.4217) ccw
  line L136 (9.6682, -142.9205) -> (10.3166, -142.8751)
  arc A544 (10.3166, -142.8751) -> (10.7817, -142.3808) centre (10.2817, -142.3763) ccw
  arc A545 (12.2887, -140.4602) -> (10.7817, -142.3808) centre (12.7816, -142.3985) ccw
  arc A546 (14.1063, -142.0899) -> (12.2887, -140.4602) centre (12.1398, -142.4546) ccw
  arc A547 (14.1063, -142.0899) -> (14.6501, -142.496) centre (14.5979, -141.9987) ccw
  line L137 (14.6501, -142.496) -> (15.2966, -142.428)
  arc A548 (15.2966, -142.428) -> (15.7441, -141.9177) centre (15.2443, -141.9308) ccw
  arc A549 (17.1832, -139.9458) -> (15.7441, -141.9177) centre (17.7435, -141.8657) ccw
  arc A550 (19.0565, -141.511) -> (17.1832, -139.9458) centre (17.104, -141.9442) ccw
  arc A551 (19.0565, -141.511) -> (19.6143, -141.8979) centre (19.5447, -141.4028) ccw
  line L138 (19.6143, -141.8979) -> (20.2579, -141.8074)
  arc A552 (20.2579, -141.8074) -> (20.6874, -141.2818) centre (20.1883, -141.3123) ccw
  arc A553 (22.0567, -139.2608) -> (20.6874, -141.2818) centre (22.6837, -141.16) ccw
  arc A554 (23.9836, -140.7598) -> (22.0567, -139.2608) centre (22.0474, -141.2608) ccw
  arc A555 (23.9836, -140.7598) -> (24.5545, -141.1269) centre (24.4676, -140.6345) ccw
  line L139 (24.5545, -141.1269) -> (25.1946, -141.014)
  arc A556 (25.1946, -141.014) -> (25.6055, -140.4738) centre (25.1078, -140.5216) ccw
  arc A557 (26.9034, -138.4062) -> (25.6055, -140.4738) centre (27.5963, -140.2824) ccw
  arc A558 (28.8814, -139.837) -> (26.9034, -138.4062) centre (26.9639, -140.4053) ccw
  arc A559 (28.8814, -139.837) -> (29.4648, -140.184) centre (29.3608, -139.6949) ccw
  line L140 (29.4648, -140.184) -> (30.1006, -140.0489)
  arc A560 (30.1006, -140.0489) -> (30.4923, -139.4946) centre (29.9966, -139.5598) ccw
  arc A561 (31.7174, -137.383) -> (30.4923, -139.4946) centre (32.4753, -139.2338) ccw
  arc A562 (33.7441, -138.7439) -> (31.7174, -137.383) centre (31.8475, -139.3787) ccw
  arc A563 (33.7441, -138.7439) -> (34.3392, -139.0703) centre (34.2182, -138.5852) ccw
  line L141 (34.3392, -139.0703) -> (34.9699, -138.9131)
  arc A564 (34.9699, -138.9131) -> (35.3421, -138.3455) centre (34.8489, -138.4279) ccw
  arc A565 (36.4926, -136.1924) -> (35.3421, -138.3455) centre (37.3147, -138.0156) ccw
  arc A566 (38.5656, -137.4817) -> (36.4926, -136.1924) centre (36.6924, -138.1824) ccw
  arc A567 (38.5656, -137.4817) -> (39.1717, -137.7872) centre (39.0339, -137.3065) ccw
  line L142 (39.1717, -137.7872) -> (39.7966, -137.608)
  arc A568 (39.7966, -137.608) -> (40.1487, -137.0278) centre (39.6587, -137.1274) ccw
  arc A569 (41.2235, -134.8358) -> (40.1487, -137.0278) centre (42.1086, -136.6293) ccw
  arc A570 (43.3402, -136.052) -> (41.2235, -134.8358) centre (41.4925, -136.8177) ccw
  arc A571 (43.3402, -136.052) -> (43.9566, -136.3362) centre (43.8021, -135.8606) ccw
  line L143 (43.9566, -136.3362) -> (44.5748, -136.1353)
  arc A572 (44.5748, -136.1353) -> (44.9065, -135.5431) centre (44.4203, -135.6598) ccw
  arc A573 (45.904, -133.315) -> (44.9065, -135.5431) centre (46.8513, -135.0765) ccw
  arc A574 (48.0619, -134.4566) -> (45.904, -133.315) centre (46.2421, -135.2862) ccw
  arc A575 (48.0619, -134.4566) -> (48.6879, -134.719) centre (48.5169, -134.2492) ccw
  line L144 (48.6879, -134.719) -> (49.2987, -134.4967)
  arc A576 (49.2987, -134.4967) -> (49.6095, -133.8933) centre (49.1277, -134.0269) ccw
  arc A577 (50.5287, -131.6318) -> (49.6095, -133.8933) centre (51.5368, -133.3591) ccw
  arc A578 (52.7251, -132.6974) -> (50.5287, -131.6318) centre (50.9353, -133.59) ccw
  arc A579 (52.7251, -132.6974) -> (53.3598, -132.9378) centre (53.1725, -132.4742) ccw
  line L145 (53.3598, -132.9378) -> (53.9625, -132.6943)
  arc A580 (53.9625, -132.6943) -> (54.2521, -132.0804) centre (53.7752, -132.2307) ccw
  arc A581 (55.0918, -129.7882) -> (54.2521, -132.0804) centre (56.1596, -131.4793) ccw
  arc A582 (57.324, -130.7764) -> (55.0918, -129.7882) centre (55.5665, -131.731) ccw
  arc A583 (57.324, -130.7764) -> (57.9668, -130.9946) centre (57.7634, -130.5378) ccw
  line L146 (57.9668, -130.9946) -> (58.5606, -130.7302)
  arc A584 (58.5606, -130.7302) -> (58.8286, -130.1066) centre (58.3572, -130.2734) ccw
  arc A585 (59.5878, -127.7864) -> (58.8286, -130.1066) centre (60.7139, -129.4392) ccw
  arc A586 (61.8532, -128.6962) -> (59.5878, -127.7864) centre (60.13, -129.7115) ccw
  arc A587 (61.8532, -128.6962) -> (62.5031, -128.8918) centre (62.2839, -128.4424) ccw
  line L147 (62.5031, -128.8918) -> (63.0873, -128.6068)
  arc A588 (63.0873, -128.6068) -> (63.3334, -127.9742) centre (62.8682, -128.1574) ccw
  arc A589 (64.0112, -125.629) -> (63.3334, -127.9742) centre (65.1943, -127.2415) ccw
  arc A590 (66.3069, -126.4592) -> (64.0112, -125.629) centre (64.6203, -127.534) ccw
  arc A591 (66.3069, -126.4592) -> (66.9633, -126.6319) centre (66.7286, -126.1905) ccw
  line L148 (66.9633, -126.6319) -> (67.5372, -126.3268)
  arc A592 (67.5372, -126.3268) -> (67.761, -125.686) centre (67.3025, -125.8853) ccw
  arc A593 (68.3566, -123.3185) -> (67.761, -125.686) centre (69.5953, -124.8887) ccw
  arc A594 (70.6799, -124.068) -> (68.3566, -123.3185) centre (69.0318, -125.2011) ccw
  arc A595 (70.6799, -124.068) -> (71.3419, -124.2178) centre (71.0919, -123.7848) ccw
  line L149 (71.3419, -124.2178) -> (71.9048, -123.8928)
  arc A596 (71.9048, -123.8928) -> (72.1061, -123.2446) centre (71.6548, -123.4598) ccw
  arc A597 (72.6187, -120.8578) -> (72.1061, -123.2446) centre (73.9114, -122.3838) ccw
  arc A598 (74.9667, -121.5258) -> (72.6187, -120.8578) centre (73.3592, -122.7156) ccw
  arc A599 (74.9667, -121.5258) -> (75.6336, -121.6523) centre (75.3686, -121.2283) ccw
  line L150 (75.6336, -121.6523) -> (76.1848, -121.3079)
  arc A600 (76.1848, -121.3079) -> (76.3634, -120.653) centre (75.9199, -120.8839) ccw
  arc A601 (76.7923, -118.2498) -> (76.3634, -120.653) centre (78.1375, -119.7298) ccw
  arc A602 (79.1623, -118.8354) -> (76.7923, -118.2498) centre (77.5972, -120.0807) ccw
  arc A603 (79.1623, -118.8354) -> (79.8331, -118.9387) centre (79.5535, -118.5241) ccw
  line L151 (79.8331, -118.9387) -> (80.372, -118.5752)
  arc A604 (80.372, -118.5752) -> (80.5276, -117.9145) centre (80.0924, -118.1607) ccw
  arc A605 (80.8724, -115.4978) -> (80.5276, -117.9145) centre (82.2684, -116.9299) ccw
  arc A606 (83.2613, -116.0003) -> (80.8724, -115.4978) centre (81.7407, -117.2994) ccw
  arc A607 (83.2613, -116.0003) -> (83.9354, -116.0801) centre (83.6415, -115.6756) ccw
  line L152 (83.9354, -116.0801) -> (84.4612, -115.698)
  arc A608 (84.4612, -115.698) -> (84.5937, -115.0323) centre (84.1673, -115.2935) ccw
  arc A609 (84.8539, -112.605) -> (84.5937, -115.0323) centre (86.2991, -113.9875) ccw
  arc A610 (87.259, -113.0239) -> (84.8539, -112.605) centre (85.7846, -114.3753) ccw
  arc A611 (87.259, -113.0239) -> (87.9354, -113.08) centre (87.6276, -112.686) ccw
  line L153 (87.9354, -113.08) -> (88.4476, -112.6799)
  arc A612 (88.4476, -112.6799) -> (88.5567, -112.01) centre (88.1398, -112.2859) ccw
  arc A613 (88.7321, -109.575) -> (88.5567, -112.01) centre (90.2247, -110.9063) ccw
  arc A614 (91.1503, -109.9097) -> (88.7321, -109.575) centre (89.724, -111.3118) ccw
  arc A615 (91.1503, -109.9097) -> (91.8283, -109.9423) centre (91.5069, -109.5592) ccw
  line L154 (91.8283, -109.9423) -> (92.3262, -109.5244)
  arc A616 (92.3262, -109.5244) -> (92.4119, -108.8511) centre (92.0048, -109.1414) ccw
  arc A617 (92.5022, -106.4116) -> (92.4119, -108.8511) centre (94.0403, -107.6899) ccw
  arc A618 (94.9306, -106.6617) -> (92.5022, -106.4116) centre (93.554, -108.1126) ccw
  arc A619 (94.9306, -106.6617) -> (95.6092, -106.6705) centre (95.2747, -106.299) ccw
  line L155 (95.6092, -106.6705) -> (96.0923, -106.2356)
  arc A620 (96.0923, -106.2356) -> (96.1544, -105.5597) centre (95.7577, -105.864) ccw
  arc A621 (96.1595, -103.1185) -> (96.1544, -105.5597) centre (97.7413, -104.3424) ccw
  arc A622 (98.5952, -103.2837) -> (96.1595, -103.1185) centre (97.2701, -104.7818) ccw
  arc A623 (98.5952, -103.2837) -> (99.2737, -103.2688) centre (98.9264, -102.9092) ccw
  line L156 (99.2737, -103.2688) -> (99.7413, -102.8173)
  arc A624 (99.7413, -102.8173) -> (99.7798, -102.1396) centre (99.394, -102.4576) ccw
  arc A625 (99.6997, -99.6997) -> (99.7798, -102.1396) centre (101.3233, -100.8677) ccw
  arc A626 (102.1396, -99.7798) -> (99.6997, -99.6997) centre (100.8677, -101.3233) ccw
  arc A627 (102.1396, -99.7798) -> (102.8173, -99.7413) centre (102.4576, -99.394) ccw
  line L157 (102.8173, -99.7413) -> (103.2688, -99.2737)
  arc A628 (103.2688, -99.2737) -> (103.2837, -98.5952) centre (102.9092, -98.9264) ccw
  arc A629 (103.1185, -96.1595) -> (103.2837, -98.5952) centre (104.7818, -97.2701) ccw
  arc A630 (105.5597, -96.1544) -> (103.1185, -96.1595) centre (104.3424, -97.7413) ccw
  arc A631 (105.5597, -96.1544) -> (106.2356, -96.0923) centre (105.864, -95.7577) ccw
  line L158 (106.2356, -96.0923) -> (106.6705, -95.6092)
  arc A632 (106.6705, -95.6092) -> (106.6617, -94.9306) centre (106.299, -95.2747) ccw
  arc A633 (106.4116, -92.5022) -> (106.6617, -94.9306) centre (108.1126, -93.554) ccw
  arc A634 (108.8511, -92.4119) -> (106.4116, -92.5022) centre (107.6899, -94.0403) ccw
  arc A635 (108.8511, -92.4119) -> (109.5244, -92.3262) centre (109.1414, -92.0048) ccw
  line L159 (109.5244, -92.3262) -> (109.9423, -91.8283)
  arc A636 (109.9423, -91.8283) -> (109.9097, -91.1503) centre (109.5592, -91.5069) ccw
  arc A637 (109.575, -88.7321) -> (109.9097, -91.1503) centre (111.3118, -89.724) ccw
  arc A638 (112.01, -88.5567) -> (109.575, -88.7321) centre (110.9063, -90.2247) ccw
  arc A639 (112.01, -88.5567) -> (112.6799, -88.4476) centre (112.2859, -88.1398) ccw
  line L160 (112.6799, -88.4476) -> (113.08, -87.9354)
  arc A640 (113.08, -87.9354) -> (113.0239, -87.259) centre (112.686, -87.6276) ccw
  arc A641 (112.605, -84.8539) -> (113.0239, -87.259) centre (114.3753, -85.7846) ccw
  arc A642 (115.0323, -84.5937) -> (112.605, -84.8539) centre (113.9875, -86.2991) ccw
  arc A643 (115.0323, -84.5937) -> (115.698, -84.4612) centre (115.2935, -84.1673) ccw
  line L161 (115.698, -84.4612) -> (116.0801, -83.9354)
  arc A644 (116.0801, -83.9354) -> (116.0003, -83.2613) centre (115.6756, -83.6415) ccw
  arc A645 (115.4978, -80.8724) -> (116.0003, -83.2613) centre (117.2994, -81.7407) ccw
  arc A646 (117.9145, -80.5276) -> (115.4978, -80.8724) centre (116.9299, -82.2684) ccw
  arc A647 (117.9145, -80.5276) -> (118.5752, -80.372) centre (118.1607, -80.0924) ccw
  line L162 (118.5752, -80.372) -> (118.9387, -79.8331)
  arc A648 (118.9387, -79.8331) -> (118.8354, -79.1623) centre (118.5241, -79.5535) ccw
  arc A649 (118.2498, -76.7923) -> (118.8354, -79.1623) centre (120.0807, -77.5972) ccw
  arc A650 (120.653, -76.3634) -> (118.2498, -76.7923) centre (119.7298, -78.1375) ccw
  arc A651 (120.653, -76.3634) -> (121.3079, -76.1848) centre (120.8839, -75.9199) ccw
  line L163 (121.3079, -76.1848) -> (121.6523, -75.6336)
  arc A652 (121.6523, -75.6336) -> (121.5258, -74.9667) centre (121.2283, -75.3686) ccw
  arc A653 (120.8578, -72.6187) -> (121.5258, -74.9667) centre (122.7156, -73.3592) ccw
  arc A654 (123.2446, -72.1061) -> (120.8578, -72.6187) centre (122.3838, -73.9114) ccw
  arc A655 (123.2446, -72.1061) -> (123.8928, -71.9048) centre (123.4598, -71.6548) ccw
  line L164 (123.8928, -71.9048) -> (124.2178, -71.3419)
  arc A656 (124.2178, -71.3419) -> (124.068, -70.6799) centre (123.7848, -71.0919) ccw
  arc A657 (123.3185, -68.3566) -> (124.068, -70.6799) centre (125.2011, -69.0318) ccw
  arc A658 (125.686, -67.761) -> (123.3185, -68.3566) centre (124.8887, -69.5953) ccw
  arc A659 (125.686, -67.761) -> (126.3268, -67.5372) centre (125.8853, -67.3025) ccw
  line L165 (126.3268, -67.5372) -> (126.6319, -66.9633)
  arc A660 (126.6319, -66.9633) -> (126.4592, -66.3069) centre (126.1905, -66.7286) ccw
  arc A661 (125.629, -64.0112) -> (126.4592, -66.3069) centre (127.534, -64.6203) ccw
  arc A662 (127.9742, -63.3334) -> (125.629, -64.0112) centre (127.2415, -65.1943) ccw
  arc A663 (127.9742, -63.3334) -> (128.6068, -63.0873) centre (128.1574, -62.8682) ccw
  line L166 (128.6068, -63.0873) -> (128.8918, -62.5031)
  arc A664 (128.8918, -62.5031) -> (128.6962, -61.8532) centre (128.4424, -62.2839) ccw
  arc A665 (127.7864, -59.5878) -> (128.6962, -61.8532) centre (129.7115, -60.13) ccw
  arc A666 (130.1066, -58.8286) -> (127.7864, -59.5878) centre (129.4392, -60.7139) ccw
  arc A667 (130.1066, -58.8286) -> (130.7302, -58.5606) centre (130.2734, -58.3572) ccw
  line L167 (130.7302, -58.5606) -> (130.9946, -57.9668)
  arc A668 (130.9946, -57.9668) -> (130.7764, -57.324) centre (130.5378, -57.7634) ccw
  arc A669 (129.7882, -55.0918) -> (130.7764, -57.324) centre (131.731, -55.5665) ccw
  arc A670 (132.0804, -54.2521) -> (129.7882, -55.0918) centre (131.4793, -56.1596) ccw
  arc A671 (132.0804, -54.2521) -> (132.6943, -53.9625) centre (132.2307, -53.7752) ccw
  line L168 (132.6943, -53.9625) -> (132.9378, -53.3598)
  arc A672 (132.9378, -53.3598) -> (132.6974, -52.7251) centre (132.4742, -53.1725) ccw
  arc A673 (131.6318, -50.5287) -> (132.6974, -52.7251) centre (133.59, -50.9353) ccw
  arc A674 (133.8933, -49.6095) -> (131.6318, -50.5287) centre (133.3591, -51.5368) ccw
  arc A675 (133.8933, -49.6095) -> (134.4967, -49.2987) centre (134.0269, -49.1277) ccw
  line L169 (134.4967, -49.2987) -> (134.719, -48.6879)
  arc A676 (134.719, -48.6879) -> (134.4566, -48.0619) centre (134.2492, -48.5169) ccw
  arc A677 (133.315, -45.904) -> (134.4566, -48.0619) centre (135.2862, -46.2421) ccw
  arc A678 (135.5431, -44.9065) -> (133.315, -45.904) centre (135.0765, -46.8513) ccw
  arc A679 (135.5431, -44.9065) -> (136.1353, -44.5748) centre (135.6598, -44.4203) ccw
  line L170 (136.1353, -44.5748) -> (136.3362, -43.9566)
  arc A680 (136.3362, -43.9566) -> (136.052, -43.3402) centre (135.8606, -43.8021) ccw
  arc A681 (134.8358, -41.2235) -> (136.052, -43.3402) centre (136.8177, -41.4925) ccw
  arc A682 (137.0278, -40.1487) -> (134.8358, -41.2235) centre (136.6293, -42.1086) ccw
  arc A683 (137.0278, -40.1487) -> (137.608, -39.7966) centre (137.1274, -39.6587) ccw
  line L171 (137.608, -39.7966) -> (137.7872, -39.1717)
  arc A684 (137.7872, -39.1717) -> (137.4817, -38.5656) centre (137.3065, -39.0339) ccw
  arc A685 (136.1924, -36.4926) -> (137.4817, -38.5656) centre (138.1824, -36.6924) ccw
  arc A686 (138.3455, -35.3421) -> (136.1924, -36.4926) centre (138.0156, -37.3147) ccw
  arc A687 (138.3455, -35.3421) -> (138.9131, -34.9699) centre (138.4279, -34.8489) ccw
  line L172 (138.9131, -34.9699) -> (139.0703, -34.3392)
  arc A688 (139.0703, -34.3392) -> (138.7439, -33.7441) centre (138.5852, -34.2182) ccw
  arc A689 (137.383, -31.7174) -> (138.7439, -33.7441) centre (139.3787, -31.8475) ccw
  arc A690 (139.4946, -30.4923) -> (137.383, -31.7174) centre (139.2338, -32.4753) ccw
  arc A691 (139.4946, -30.4923) -> (140.0489, -30.1006) centre (139.5598, -29.9966) ccw
  line L173 (140.0489, -30.1006) -> (140.184, -29.4648)
  arc A692 (140.184, -29.4648) -> (139.837, -28.8814) centre (139.6949, -29.3608) ccw
  arc A693 (138.4062, -26.9034) -> (139.837, -28.8814) centre (140.4053, -26.9639) ccw
  arc A694 (140.4738, -25.6055) -> (138.4062, -26.9034) centre (140.2824, -27.5963) ccw
  arc A695 (140.4738, -25.6055) -> (141.014, -25.1946) centre (140.5216, -25.1078) ccw
  line L174 (141.014, -25.1946) -> (141.1269, -24.5545)
  arc A696 (141.1269, -24.5545) -> (140.7598, -23.9836) centre (140.6345, -24.4676) ccw
  arc A697 (139.2608, -22.0567) -> (140.7598, -23.9836) centre (141.2608, -22.0474) ccw
  arc A698 (141.2818, -20.6874) -> (139.2608, -22.0567) centre (141.16, -22.6837) ccw
  arc A699 (141.2818, -20.6874) -> (141.8074, -20.2579) centre (141.3123, -20.1883) ccw
  line L175 (141.8074, -20.2579) -> (141.8979, -19.6143)
  arc A700 (141.8979, -19.6143) -> (141.511, -19.0565) centre (141.4028, -19.5447) ccw
  arc A701 (139.9458, -17.1832) -> (141.511, -19.0565) centre (141.9442, -17.104) ccw
  arc A702 (141.9177, -15.7441) -> (139.9458, -17.1832) centre (141.8657, -17.7435) ccw
  arc A703 (141.9177, -15.7441) -> (142.428, -15.2966) centre (141.9308, -15.2443) ccw
  line L176 (142.428, -15.2966) -> (142.496, -14.6501)
  arc A704 (142.496, -14.6501) -> (142.0899, -14.1063) centre (141.9987, -14.5979) ccw
  arc A705 (140.4602, -12.2887) -> (142.0899, -14.1063) centre (142.4546, -12.1398) ccw
  arc A706 (142.3808, -10.7817) -> (140.4602, -12.2887) centre (142.3985, -12.7816) ccw
  arc A707 (142.3808, -10.7817) -> (142.8751, -10.3166) centre (142.3763, -10.2817) ccw
  line L177 (142.8751, -10.3166) -> (142.9205, -9.6682)
  arc A708 (142.9205, -9.6682) -> (142.4956, -9.1388) centre (142.4217, -9.6333) ccw
  arc A709 (140.8035, -7.3792) -> (142.4956, -9.1388) centre (142.7915, -7.1608) ccw
  arc A710 (142.6703, -5.8061) -> (140.8035, -7.3792) centre (142.7578, -7.8042) ccw
  arc A711 (142.6703, -5.8061) -> (143.1481, -5.324) centre (142.6484, -5.3066) ccw
  line L178 (143.1481, -5.324) -> (143.1708, -4.6744)
  arc A712 (143.1708, -4.6744) -> (142.7278, -4.1602) centre (142.6711, -4.657) ccw
  arc A713 (140.9752, -2.4607) -> (142.7278, -4.1602) centre (142.9545, -2.1731) ccw
  arc A714 (142.786, -0.8235) -> (140.9752, -2.4607) centre (142.9432, -2.8173) ccw
  arc A715 (142.786, -0.8235) -> (143.2467, -0.325) centre (142.7467, -0.325) ccw
  line L179 (143.2467, -0.325) -> (143.2467, 0.325)
  arc A716 (143.2467, 0.325) -> (142.786, 0.8235) centre (142.7467, 0.325) ccw
  arc A717 (140.9752, 2.4607) -> (142.786, 0.8235) centre (142.9432, 2.8173) ccw
  arc A718 (142.7278, 4.1602) -> (140.9752, 2.4607) centre (142.9545, 2.1731) ccw